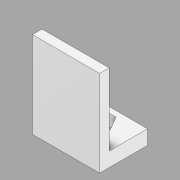
# Autodesk Inventor part: uchwyt_krancowka_alternatywa_2
Saved by Autodesk Inventor 2021 (Build 250183000, 183)
## iProperties
Created: 2022-09-08
Part Number: uchwyt_krancowka_alternatywa_2
Material: Generic
Document SubType Name: Modeling
Designer: agnpi
Density: 1 g/cm^3
Appearance: Snow
Author: agnpi
Autodesk Inventor part; units mm, degrees
ref_plane "YZ Plane" through (0, 0, 0) normal (1, 0, 0) x (0, 1, 0)
ref_plane "XZ Plane" through (0, 0, 0) normal (0, 1, 0) x (-1, 0, 0)
ref_plane "XY Plane" through (0, 0, 0) normal (0, 0, 1) x (1, 0, 0)
sketch "Sketch1" plane through (0, 0, 0) normal (0, 1, 0) x (-1, 0, 0)
  line L0 (9.8, 0) -> (-9.8, 0) projected
  line L1 (0, -7) -> (0, 7) projected
  line L2 (-7, 5) -> (7, 5)
  line L3 (7, 5) -> (7, -5)
  line L4 (7, -5) -> (-7, -5)
  line L5 (-7, -5) -> (-7, 5)
  line L6 (-7, 5) -> (7, -5) construction
  line L7 (7, 5) -> (-7, -5) construction
  point P0 (0, 0)
  dimension "d0" = 14
  dimension "d1" = 10
  constraints: 12 end point, 2 midpoint, 2 parallel, 1 horizontal, 1 perpendicular
  measures "d0" distance of L3.end L4.end
  measures "d1" distance of L2.end L3.end
extrude "Extrusion1" add sketch "Sketch1" along normal blind 3
sketch "Sketch2" plane through (0, 3, 0) normal (0, 1, 0) x (1, 0, 0)
  line L0 (-7, 5) -> (-7, -5) projected
  line L1 (7, -5) -> (7, 5) projected
  line L2 (-7, -5) -> (7, -5)
  line L3 (7, -5) -> (7, -3)
  line L4 (7, -3) -> (-7, -3)
  line L5 (-7, -3) -> (-7, -5)
  point P0 (0, 0)
  point P1 (7, -5)
  point P2 (-7, -3)
  dimension "d4" = 2
  constraints: 8 end point, 2 parallel, 1 horizontal, 1 perpendicular, 1 point on line
  measures "d4" distance between parallel lines of L2 L4
extrude "Extrusion2" add sketch "Sketch2" along normal blind 15
sketch "Sketch4" plane through (0, 3, 0) normal (0, 1, 0) x (1, 0, 0)
  line L0 (1.625, -1.8146) -> (-1.625, -1.8146)
  line L1 (-1.625, -1.8146) -> (-3.25, 1)
  line L2 (-3.25, 1) -> (-1.625, 3.8146)
  line L3 (-1.625, 3.8146) -> (1.625, 3.8146)
  line L4 (1.625, 3.8146) -> (3.25, 1)
  line L5 (3.25, 1) -> (1.625, -1.8146)
  line L6 (7, 5) -> (-7, 5) projected
  line L7 (-7, 5) -> (-7, -3) projected
  point P0 (0, 0)
  point P1 (0, 1)
  dimension "d8" = 6.5
  dimension "d9" = 3.25
  dimension "d10" = 4
  dimension "d11" = 7
  constraints: 12 end point, 13 other
  measures "d8" distance of L0.start L2.end
  measures "d9" distance of L2.end L3.end
  measures "d10" distance from line of L6 point (0, 1)
  measures "d11" distance from line of L7 point (0, 1)
extrude "Extrusion3" cut sketch "Sketch4" against normal blind 2.5
sketch "Sketch5" plane through (0, 0.5, 0) normal (0, 1, 0) x (1, 0, 0)
  line L0 (-3.25, 1) -> (-1.625, 3.8146) projected
  line L1 (-1.625, 3.8146) -> (1.625, 3.8146) projected
  point P0 (0, 0)
  point P1 (0.008, 1.0001)
  dimension "d21" = 2.8215
  dimension "d22" = 2.8145
  measures "d21" distance from line of L0 point (0.008, 1)
  measures "d22" distance from line of L1 point (0.008, 1)
hole "Hole1" at (0.008, 0.5, -1.0001) direction (0, -1, 0) diameter 3 end through all
body "Solid1"
